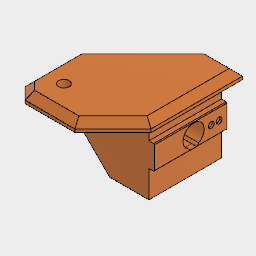
rambo_base_upper_mount v2 (Autodesk Fusion 360 design; units mm, degrees)
Autodesk Fusion 360 part; units mm, degrees
sketch "base" plane through (0, 0, 0) normal (0, 0, 1) x (1, 0, 0)
  line L0 (0, 0) -> (20, 0)
  line L1 (20, 0) -> (20, 33.05)
  line L2 (20, 33.05) -> (14.5, 33.05)
  line L3 (14.5, 33.05) -> (14.5, 14.55)
  line L4 (14.5, 16.55) -> (0, 16.55)
  line L5 (0, 16.55) -> (0, 0)
  line L6 (0, 14.55) -> (20, 14.55)
  line L7 (6, 9.9311) -> (3.375, 8.4155)
  line L8 (3.375, 8.4155) -> (3.375, 5.3845)
  line L9 (3.375, 5.3845) -> (6, 3.8689)
  line L10 (6, 3.8689) -> (8.625, 5.3845)
  line L11 (8.625, 5.3845) -> (8.625, 8.4155)
  line L12 (8.625, 8.4155) -> (6, 9.9311)
  circle A0 centre (6, 6.9) radius 1.35
  line L13 (16.5, 33.05) -> (0, 16.55)
  line L14 (20, 4.292) -> (15.708, 0)
  line L15 (20, 4.292) -> (25.4, 9.692)
  line L16 (25.4, 9.692) -> (25.4, 33.05)
  line L17 (25.4, 33.05) -> (20, 33.05)
  circle A1 centre (6, 6.9) radius 2.625 construction
  line L18 (14.5, 24.55) -> (20, 24.55) construction
  point P0 (6, 6.9)
  dimension "d2037" = 6.9
  dimension "d2040" = 14
  dimension "d2042" = 2.7
  dimension "d2072" = 0
  dimension "d2073" = 0
  dimension "d2074" = 0
  dimension "d2075" = 0
  dimension "d2087" = 5.4
  dimension "d1" = 5.25
  dimension "d4" = 7.65
  dimension "d5" = 2
  dimension "d19" = 8
  dimension "d20" = 8.5
  dimension "d26" = 9.708
  dimension "d28" = 45
  dimension "d30" = 6
  dimension "d31" = 5.5
  measures "d2037" distance of L0.start A0.centre
  measures "d2040" distance of L0.end P0
  measures "d2042" diameter of A0
  measures "d2087" distance of L1.end L16.end
  measures "d1" diameter of A1
  measures "d4" distance of P0 L6.start
  measures "d5" distance of L4.end L6.start
  measures "d19" distance of L4.start L18.start
  measures "d20" distance of L2.end L18.start
  measures "d26" distance of P0 L14.end
  measures "d28" angle of L0 L14
  measures "d30" distance of L0.start A0.centre
  measures "d31" distance of L1.end L2.end
extrude "Extrude1" add sketch "base" along normal blind 2.5 contours L0 L1 L5 L6 L14 | L3 L4 L5 L6 | L3 L4 L13 | L1 L2 L3 L6 L13 | L7 L8 L9 L10 L11 L12
extrude "Extrude2" add sketch "base" against normal blind 20 contours L1 L2 L3 L6 L13
extrude "Extrude3" add sketch "base" against normal up to surface (20 mm away) contours L3 L4 L5 L6
extrude "Extrude4" add sketch "base" against normal blind 2.8 contours L7 L8 L9 L10 L11 L12
extrude "Extrude10" add sketch "base" along normal up to surface (2.5 mm away) contours L1 L15 L16 L17
extrude "Extrude7" add 1 faces at (9.6667, 21.3833, 0) along direction (0, 0, -1) blind 2.5
sketch "rail_profile" plane through (0, 33.05, 0) normal (0, 1, 0) x (-1, 0, 0)
  line L0 (-16.5, -20) -> (-16.5, 2.5)
  line L1 (-16.5, 2.5) -> (-25.4, 2.5)
  line L2 (-25.4, 2.5) -> (-25.4, 0)
  line L3 (-20, -20) -> (-16.5, -20)
  line L4 (-21.4, -12.85) -> (-21.4, -7.15)
  line L5 (-21.4, -10) -> (-20, -10) construction
  line L6 (-25.4, 0) -> (-20, 0)
  line L7 (-20, 0) -> (-20, -20)
  line L8 (-20, 0) -> (-20, -20)
  line L9 (-20.225, -5.775) -> (-20, -5.775)
  line L10 (-20.225, -14.225) -> (-20, -14.225)
  line L11 (-21.2, -13.05) -> (-20, -13.05)
  line L12 (-21.2, -6.95) -> (-20, -6.95)
  arc A0 (-21.2, -6.95) -> (-21.4, -7.15) centre (-21.2, -7.15) ccw
  arc A1 (-21.4, -12.85) -> (-21.2, -13.05) centre (-21.2, -12.85) ccw
  dimension "d8" = 10
  dimension "d77" = 1.4
  dimension "d152" = 0.2
  measures "d8" distance of L6.end L5.start
  measures "d77" distance of L4 L3.start
  measures "d152" radius of A0
extrude "Extrude11" add sketch "rail_profile" against normal up to surface (18.5 mm away) contours L4 L7 L8 L11 L12 A0 A1
sketch "frame_hole" plane through (14.5, 0, 0) normal (-1, 0, 0) x (0, -1, 0)
  line L0 (-16.55, -2.5) -> (-31.05, -2.5)
  line L1 (-31.05, -20) -> (-16.55, -20)
  line L2 (-16.55, -20) -> (-16.55, -2.5)
  circle A0 centre (-24.55, -10) radius 2.7
  line L3 (-33.05, -12.85) -> (-33.05, -7.15)
  line L4 (-16.55, -20) -> (-16.55, -2.5)
  line L5 (-33.05, -10) -> (-16.55, -10) construction
  circle A1 centre (-24.55, -10) radius 5
  line L6 (-23.225, -12.3525) -> (-23.7735, -12.901)
  line L7 (-23.7735, -12.901) -> (-25.3265, -12.901)
  line L8 (-25.3265, -12.901) -> (-25.875, -12.3525)
  line L9 (-24.55, -12.901) -> (-24.55, -10) construction
  line L10 (-16.55, -20) -> (-31.05, -20)
  line L11 (-29.55, -10) -> (-29.55, -20)
  line L12 (-31.05, -2.5) -> (-31.05, -20)
  line L13 (-19.55, -10) -> (-19.55, -20)
  dimension "d15" = 5.4
  dimension "d32" = 10
  dimension "d40" = 0.201
  dimension "d41" = 45
  dimension "d42" = 45
  dimension "d43" = 2.65
  dimension "d127" = 3
  measures "d15" diameter of A0
  measures "d32" diameter of A1
  measures "d40" distance of A0 L7
  measures "d41" angle of L6 L7
  measures "d42" angle of L7 L8
  measures "d43" distance of L6.start L8.end
  measures "d127" distance of L1.end L13.end
extrude "Extrude12" cut sketch "frame_hole" against normal blind 17 contours A0 | A0 L6 L7 L8
extrude "Extrude14" cut sketch "frame_hole" against normal blind 2 contours L1 A1 L10 L11 L13 | A1 | A0 L6 L7 L8
sketch "rambo_cover_tolerance" plane through (0, 0, 0) normal (-1, 0, 0) x (0, -1, 0)
  line L0 (-14.55, 0) -> (0, 0)
  line L1 (0, 0) -> (0, 2.5)
  line L2 (0, 2.5) -> (-16.55, 2.5)
  line L3 (-16.55, 2.5) -> (-16.55, -2.5)
  line L4 (-16.55, -20) -> (-14.55, -20)
  line L5 (-14.55, -20) -> (-14.55, 0)
  line L6 (-14.55, 0) -> (-14.55, -20)
  line L7 (-14.55, 0) -> (0, 0)
  line L8 (-14.55, -0.45) -> (-14.751, -0.249)
  line L9 (-14.55, 0) -> (-14.751, 0)
  line L10 (-14.751, 0) -> (-14.751, -0.249)
  line L11 (-16.55, -2.5) -> (-16.55, -20)
  dimension "d48" = 135
  dimension "d49" = 0.45
  dimension "d50" = 0.201
  measures "d48" angle of L5 L8
  measures "d49" distance of L0.start L8.start
  measures "d50" distance of L6 L8.end
extrude "Extrude17" cut sketch "rambo_cover_tolerance" against normal blind 22.5 contours L5 L6 L8 L9 L10
chamfer "Chamfer11" distance 2.4748 angle 45 1 edges at (15.5, 32.05, -20)
sketch "better_printed_angle" plane through (0, 33.05, 0) normal (0, 1, 0) x (-1, 0, 0)
  line L0 (-16.5, -17.5252) -> (-16.5, 2.5)
  line L1 (-16.5, 2.5) -> (-25.4, 2.5)
  line L2 (-25.4, 2.5) -> (-25.4, 0)
  line L3 (-25.4, 0) -> (-20, 0)
  line L4 (-20, 0) -> (-20, -6.95)
  line L5 (-21.4, -7.15) -> (-21.4, -12.85)
  line L6 (-25.4, 0) -> (-20, 0)
  line L7 (-20, 0) -> (-20, -6.95)
  line L8 (-20, 0) -> (-20, 0.201)
  line L9 (-20, 0.201) -> (-20.225, 0.201)
  line L10 (-20.225, 0.201) -> (-20.225, 0)
  line L11 (-19.9999, -20) -> (-16.5, -17.5252)
  line L12 (-20, -20) -> (-19.9999, -20)
  line L13 (-20, -6.95) -> (-21.2, -6.95)
  arc A0 (-21.2, -6.95) -> (-21.4, -7.15) centre (-21.2, -7.15) ccw
  arc A1 (-21.4, -12.85) -> (-21.2, -13.05) centre (-21.2, -12.85) ccw
  line L14 (-21.2, -13.05) -> (-20, -13.05)
  line L15 (-20, -13.05) -> (-20, -20)
  dimension "d107" = 0.225
  dimension "d108" = 0.201
  measures "d107" distance of L8.end L9.end
  measures "d108" distance of L9.end L10.end
extrude "Extrude22" cut sketch "better_printed_angle" against normal up to surface (18.2 mm away) contours L3 L6 L8 L9 L10
sketch "mk_type" plane through (21.4, 0, 0) normal (1, 0, 0) x (0, 1, 0)
  line L0 (25.875, -12.3525) -> (25.3775, -12.85)
  line L1 (23.7225, -12.85) -> (23.225, -12.3525)
  arc A0 (25.875, -12.3525) -> (23.225, -12.3525) centre (24.55, -10) ccw
  line L2 (14.55, -7.15) -> (14.55, -12.85)
  line L3 (33.05, -12.85) -> (33.05, -7.15)
  line L4 (33.05, -12.85) -> (33.05, -7.15)
  line L5 (33.05, -10) -> (29.05, -10) construction
  circle A1 centre (29.05, -10) radius 0.75
  circle A2 centre (31.05, -10) radius 0.75
  line L6 (25.3775, -12.85) -> (33.05, -12.85)
  line L7 (33.05, -7.15) -> (14.55, -7.15)
  line L8 (14.55, -12.85) -> (23.7225, -12.85)
  dimension "d101" = 1.5
  dimension "d102" = 1.5
  dimension "d103" = 2
  dimension "d104" = 2
  measures "d101" diameter of A1
  measures "d102" diameter of A2
  measures "d103" distance of L5.end A2.centre
  measures "d104" distance of L5.start A2.centre
extrude "Extrude23" cut sketch "mk_type" against normal blind 0.5 contours A1 | A2
chamfer "Chamfer3" distance 3 angle 45 1 edges at (0, 0, 1.25)
chamfer "Chamfer15" distance 1.7 angle 45 7 edges at (8.25, 24.8, 2.5) (0, 9.775, 2.5) (1.5, 1.5, 2.5) (9.354, 0, 2.5) (20.554, 4.846, 2.5) (25.4, 21.371, 2.5) (20.95, 33.05, 2.5)
chamfer "Chamfer6" distance 0.3 angle 45 6 edges at (3.375, 6.9, -2.8) (4.6875, 9.1733, -2.8) (7.3125, 9.1733, -2.8) (8.625, 6.9, -2.8) (7.3125, 4.6267, -2.8) (4.6875, 4.6267, -2.8)
chamfer "Chamfer8" distance 1.5 angle 45 1 edges at (14.5, 23.8, -2.5)
chamfer "Chamfer9" distance 10 angle 45 1 edges at (0, 15.55, -20)
chamfer "Chamfer10" distance 0.7 angle 45 3 edges at (5, 16.55, -15) (12.25, 16.55, -20) (0, 16.55, -6.25)
chamfer "Chamfer12" distance 2 angle 45 1 edges at (14.5, 17.7, -20)
chamfer "Chamfer13" distance 0.2 distance2 0.7 1 edges at (4.7414, 6.4118, -2.8) measured on face at (8, 6.9, -2.8)
chamfer "Chamfer14" distance 0.7 angle 45 1 edges at (0, 16.2, -2.5)
sketch "selective_infill_frame_hole" plane through (16.5, 0, 0) normal (-1, 0, 0) x (0, -1, 0)
  line L0 (-29.55, -10) -> (-29.55, -20)
  arc A0 (-23.225, -12.3525) -> (-25.875, -12.3525) centre (-24.55, -10) ccw
  line L1 (-30.55, -9.8995) -> (-29.75, -9.8995)
  line L2 (-29.75, -9.8995) -> (-29.75, -10.1005)
  line L3 (-29.75, -10.1005) -> (-30.55, -10.1005)
  line L4 (-30.55, -10.1005) -> (-30.55, -9.8995)
  line L5 (-19.35, -9.5) -> (-19.249, -9.5)
  line L6 (-19.249, -9.5) -> (-19.249, -10.5)
  line L7 (-19.249, -10.5) -> (-19.35, -10.5)
  line L8 (-19.35, -10.5) -> (-19.35, -9.5)
  line L9 (-29.75, -10) -> (-19.35, -10) construction
  arc A1 (-19.55, -10) -> (-29.55, -10) centre (-24.55, -10) ccw
  line L10 (-23.225, -12.3525) -> (-23.7735, -12.901)
  line L11 (-23.7735, -12.901) -> (-25.3265, -12.901)
  line L12 (-25.3265, -12.901) -> (-25.875, -12.3525)
  arc A2 (-23.225, -12.3525) -> (-25.875, -12.3525) centre (-24.55, -10) ccw
  line L13 (-29.55, -20) -> (-19.55, -20)
  line L14 (-19.55, -20) -> (-19.55, -10)
  line L15 (-33.05, -12.85) -> (-33.05, -7.15)
  dimension "d81" = 0.101
  dimension "d82" = 1
  dimension "d85" = 0.201
  dimension "d128" = 2.5
  dimension "d129" = 2.5
  measures "d81" distance of L6.end L7.end
  measures "d82" distance of L5.start L7.end
  measures "d85" distance of L1.start L3.end
  measures "d128" distance of L4 L15
  measures "d129" distance of L2 A2
extrude "Extrude20" cut sketch "selective_infill_frame_hole" against normal blind 0.101 from surface at -2.5 contours L1 L2 L3 L4 | L5 L6 L7 L8
sketch "selective_infill_base" plane through (0, 0, 2.5) normal (0, 0, 1) x (-1, 0, 0)
  line L0 (-2.85, -9.3376) -> (-22.55, -29.0376)
  line L1 (-22.55, -29.0376) -> (-22.55, -28.8947)
  line L2 (-22.55, -28.8947) -> (-2.85, -9.1947)
  line L3 (-2.85, -9.1947) -> (-2.85, -9.3376)
  line L4 (-7.5376, -2.85) -> (-22.55, -17.8624)
  line L5 (-22.55, -17.8624) -> (-22.55, -18.0053)
  line L6 (-22.55, -18.0053) -> (-7.3947, -2.85)
  line L7 (-7.3947, -2.85) -> (-7.5376, -2.85)
  line L8 (-23.7, -10.3962) -> (-15.0038, -1.7)
  line L9 (-23.7, -31.35) -> (-23.7, -10.3962)
  line L10 (-17.2042, -31.35) -> (-23.7, -31.35)
  line L11 (-1.7, -15.8458) -> (-17.2042, -31.35)
  line L12 (-1.7, -3.7042) -> (-1.7, -15.8458)
  line L13 (-15.0038, -1.7) -> (-3.7042, -1.7)
  circle A0 centre (-6, -6.9) radius 1.35
  dimension "d125" = 0.101
  dimension "d126" = 0.101
  dimension "d144" = 2.5
  dimension "d145" = 2.5
  dimension "d146" = 1.15
  dimension "d147" = 1.15
  dimension "d148" = 1.15
  dimension "d151" = 1.15
  measures "d125" distance of L0 L2
  measures "d126" distance of L4 L6
  measures "d144" distance of L6 A0
  measures "d145" distance of L2 A0
  measures "d146" distance of L7 L13
  measures "d147" distance of L3 L12
  measures "d148" distance of L5 L9
  measures "d151" distance of L1 L9
extrude "Extrude24" cut sketch "selective_infill_base" against normal blind 0.201 from surface at -1.15 contours L0 L1 L2 L3 | L4 L5 L6 L7
sketch "Sketch16" plane through (0, 0, 2.5) normal (0, 0, 1) x (-1, 0, 0)
  line L0 (-0.7, -16.55) -> (-13, -16.55)
  line L1 (-20, -14.55) -> (0, -14.55)
  line L2 (-4.7426, -17.05) -> (-4.8436, -17.05)
  line L3 (-4.8436, -17.05) -> (-4.8436, -14.05)
  line L4 (-4.8436, -14.05) -> (-4.7426, -14.05)
  line L5 (-4.7426, -14.05) -> (-4.7426, -17.05)
  line L6 (-16.5, -33.05) -> (0, -16.55)
  dimension "d132" = 0.101
  dimension "d133" = 0.5
  dimension "d134" = 0.5
  dimension "d150" = 3
  measures "d132" distance of L3.end L4.end
  measures "d133" distance of L1 L4.end
  measures "d134" distance of L0 L2.start
  measures "d150" distance of L2.start L6
extrude "Extrude25" cut sketch "Sketch16" along normal mid plane 0.201 from surface at -1.25
equation "d2034 = 7.5 mm + 0.1 mm"
equation "m5_hole_dia = 5.3 mm"
equation "m5_head_dia = 10 mm"
equation "d15 = m5_hole_dia + 0.1 mm"
equation "d19 = m5_head_dia / 2 + 3 mm"
equation "d26 = ( 6 * 1.618 ) * 1 mm"
equation "d32 = m5_head_dia"
equation "layer_height = 0.2 mm"
equation "d40 = layer_height + 0.001 mm"
equation "d43 = m5_hole_dia / 2"
equation "d49 = extrusion_width"
equation "d50 = layer_height + 0.001 mm"
equation "rail_profile_width = 8.9 mm"
equation "rail_profile_height = 1.4 mm"
equation "extrusion_width = 0.45 mm"
equation "num_top_bottom = 5"
equation "num_perimeters = 3"
equation "perimeters_thickness = num_perimeters * extrusion_width - 0.1 mm"
equation "top_bottom_thickness = num_top_bottom * layer_height"
equation "d77 = rail_profile_height"
equation "d85 = layer_height + 0.001 mm"
equation "d86 = -perimeters_thickness * 2"
equation "d102 = d101"
equation "d104 = d103"
equation "d107 = extrusion_width / 2"
equation "d108 = layer_height + 0.001 mm"
equation "d119 = ( -2.5 / 2 ) * 1 mm + layer_height / 2"
equation "d120 = -layer_height - 0.001 mm"
equation "d128 = perimeters_thickness * 2"
equation "d129 = perimeters_thickness * 2"
equation "d136 = ( -2.5 / 2 ) * 1 mm"
equation "d137 = layer_height + 0.001 mm"
equation "d143 = 2.5 mm - layer_height * 4"
equation "d144 = perimeters_thickness * 2"
equation "d145 = perimeters_thickness * 2"
equation "d147 = d146"
equation "d148 = d146"
equation "d151 = d146"
